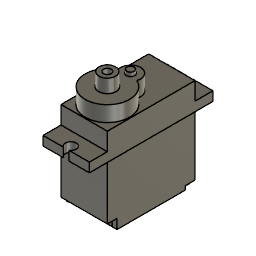
Davinki Assembly (Autodesk Fusion 360 archive; units mm, degrees)
design "Sg90Servo"
Autodesk Fusion 360 part; units mm, degrees
sketch "Sketch2" plane through (0, 0, 0) normal (0, 1, 0) x (1, 0, 0)
  line L0 (-6, -6) -> (6, -6)
  line L1 (6, -6) -> (6, 16.7)
  line L2 (6, 16.7) -> (-6, 16.7)
  line L3 (-6, 16.7) -> (-6, -6)
  line L4 (0, 0) -> (0, -6) construction
  line L5 (6, -6) -> (6, -10.65)
  line L6 (6, -10.65) -> (-6, -10.65)
  line L7 (-6, -10.65) -> (-6, -6)
  line L8 (6, 16.7) -> (6, 21.35)
  line L9 (6, 21.35) -> (-6, 21.35)
  line L10 (-6, 21.35) -> (-6, 16.7)
  line L11 (0, -10.65) -> (0, -9.45) construction
  line L12 (0, 21.35) -> (0, 20.15) construction
  circle A0 centre (0, 20.15) radius 1.4
  circle A1 centre (0, -9.45) radius 1.4
  dimension "d1" = 12
  dimension "d2" = 22.7
  dimension "d4" = 6
  dimension "d11" = 2.8
  dimension "d12" = 1.2
  dimension "d13" = 32
  constraint horizontal L0
  constraint vertical L1
  constraint horizontal L2
  constraint vertical L3
  constraint coincident L4.start origin
  constraint midpoint L0 L4.end
  constraint perpendicular L0 L4
  constraint vertical L7
  constraint horizontal L6
  constraint vertical L5
  constraint vertical L8
  constraint vertical L10
  constraint horizontal L9
  constraint equal L7 L10
  constraint midpoint L6 L11.start
  constraint perpendicular L6 L11
  constraint perpendicular L9 L12
  constraint coincident L12.end A0.centre
  constraint coincident L11.end A1.centre
  constraint equal L11 L12
  constraint equal A0 A1
  constraint midpoint L9 L12.start
  measures "d1" distance of L0.start L0.end
  measures "d2" distance of L0.start L2.end
  measures "d4" distance of L4.start L4.end
  measures "d11" diameter of A0
  measures "d12" distance of L12.start L12.end
  measures "d13" distance of L6 L9
extrude "Extrude1" add sketch "Sketch2" against normal blind 7 contours L0 L1 L2 L3 makes body 1
extrude "Extrude2" add sketch "Sketch2" along normal blind 2.4 from surface at -7 contours L0 L5 L6 L7 A1 | L2 L8 L9 L10 A0 bodies 1
extrude "Extrude3" add sketch "Sketch2" against normal blind 16.3 from surface at -7 separate body contours L0 L1 L2 L3 makes body 2
sketch "Sketch4" plane through (0, -23.3, 0) normal (0, -1, 0) x (1, 0, 0)
  line L0 (6, 6) -> (-6, 6)
  line L1 (-6, 6) -> (-6, -16.7)
  line L2 (-6, -16.7) -> (6, -16.7)
  line L3 (6, -16.7) -> (6, 6)
  circle A0 centre (4.75, -15.45) radius 1.25
  line L4 (4.75, -14.2) -> (6, -14.2)
  line L5 (3.5, -15.45) -> (3.5, -16.7)
  line L6 (-1.75, 6) -> (1.75, 6)
  line L7 (1.75, 6) -> (1.75, 4.5)
  line L8 (1.75, 4.5) -> (-1.75, 4.5)
  line L9 (-1.75, 4.5) -> (-1.75, 6)
  point P0 (0, 6)
  dimension "d20" = 2.5
  dimension "d31" = 1.5
  dimension "d32" = 3.5
  constraint tangent L3 A0
  constraint tangent L2 A0
  constraint coincident A0 L4.start
  constraint coincident L3 L4.end
  constraint tangent A0 L4
  constraint coincident A0 L5.start
  constraint coincident L2 L5.end
  constraint tangent A0 L5
  constraint perpendicular L2 L5
  constraint horizontal L4
  constraint horizontal L6
  constraint vertical L7
  constraint horizontal L8
  constraint vertical L9
  constraint midpoint L6 P0
  constraint midpoint L0 P0
  measures "d20" diameter of A0
  measures "d31" distance of L6.end L7.end
  measures "d32" distance of L7.end L8.end
ref_plane "WorkPlane1" through (0, -13.9, -5.35) normal (0, 0, 1) x (-1, 0, 0)
extrude "Extrude4" cut sketch "Sketch4" against normal blind 1 contours L3 A0 L4 | A0 | L2 L3 A0 | L2 A0 L5 bodies 2
mirror "Mirror1" about plane through (0, 0, 0) normal (1, 0, 0) of "Extrude4"
mirror "Mirror2" about plane through (0, -13.9, -5.35) normal (0, 0, 1) of "Extrude4", "Mirror1"
extrude "Extrude5" cut 2 faces at (4.75, -22.3, 4.75) (-4.75, -22.3, 4.75) along direction (0, 1, 0) blind 1.5 on bodies 2 bodies 2
chamfer "Chamfer1" distance 2.5 angle 45 1 edges at (0, -23.3, 6) tangent chain off on bodies 2
extrude "Extrude6" cut sketch "Sketch4" against normal blind 2.5 contours L0 L6 L7 L8 L9 bodies 2
sketch "Sketch3" plane through (0, 0, 0) normal (0, 1, 0) x (1, 0, 0)
  circle A0 centre (0, 0) radius 2.25
  circle A1 centre (0, 0) radius 5.75
  circle A2 centre (0, 6) radius 2.6
  line L0 (0, 6) -> (0, 0) construction
  line L1 (2.6, 6) -> (2.6, 5.1286)
  line L2 (-2.6, 6) -> (-2.6, 5.1286)
  circle A3 centre (0, 6) radius 1.1
  dimension "d5" = 4.5
  dimension "d6" = 11.5
  dimension "d7" = 5.2
  dimension "d8" = 6
  dimension "d60" = 2.2
  constraint coincident A0.centre A1.centre
  constraint coincident A2.centre L0.start
  constraint vertical L0
  constraint coincident A2 L1.start
  constraint coincident A1 L1.end
  constraint tangent A2 L1
  constraint coincident A2 L2.start
  constraint coincident A1 L2.end
  constraint tangent A2 L2
  constraint parallel L0 L2
  constraint vertical L1
  constraint concentric A2 A3
  measures "d5" diameter of A0
  measures "d6" diameter of A1
  measures "d7" diameter of A2
  measures "d8" distance of A2.centre A0.centre
  measures "d60" diameter of A3
extrude "Extrude7" add sketch "Sketch3" along normal blind 4 contours A1 A2 | A1 A2 A3 | A1 A2 A3 | A1 A3 | A1 A3 bodies 1
extrude "Extrude10" add sketch "Sketch3" along normal blind 0.9 draft -10 from surface at 4 contours A1 A3 | A1 A3 bodies 1
extrude "Extrude1'" add 1 faces at (1.1556, 0, 0.7479) along direction (0, 1, 0) blind 4 separate body on bodies 1 makes body 3 in component "Component"
extrude "Extrude2'" add 1 faces at (1.1556, 4, 0.7479) along direction (0, 1, 0) blind 3.4 draft -2 on bodies 3 bodies 3 in component "Component"
sketch "Sketch1" plane through (0, 7.4, 0) normal (0, 1, 0) x (-1, 0, 0) in component "Component"
  circle A0 centre (0, 0) radius 2.1313
  circle A1 centre (0, 0) radius 1
  dimension "d41" = 2
  constraint coincident A0.centre A1.centre
  measures "d41" diameter of A1
extrude "Extrude3'" cut sketch "Sketch1" against normal blind 3 contours A1 bodies 3 in component "Component"
sketch "Sketch5" plane through (0, -22.3, 0) normal (0, -1, 0) x (1, 0, 0)
  arc A0 (4.75, -14.2) -> (3.5, -15.45) centre (4.75, -15.45) ccw
  line L0 (3.5, -15.45) -> (3.5, -16.7)
  line L1 (3.5, -16.7) -> (6, -16.7)
  line L2 (6, -16.7) -> (6, -14.2)
  line L3 (6, -14.2) -> (4.75, -14.2)
  circle A1 centre (4.75, -15.45) radius 1
  dimension "d44" = 2
  constraint concentric A0 A1
  measures "d44" diameter of A1
extrude "Extrude8" add sketch "Sketch5" along normal blind 0.7 separate body contours A1 makes body 4
sketch "Sketch6" plane through (0, -23, 0) normal (0, -1, 0) x (1, 0, 0)
  circle A0 centre (4.75, -15.45) radius 1
  line L0 (4.5, -16.25) -> (5, -16.25)
  line L1 (5, -16.25) -> (5, -14.65)
  line L2 (5, -14.65) -> (4.5, -14.65)
  line L3 (4.5, -14.65) -> (4.5, -16.25)
  line L4 (4.5, -16.25) -> (5, -14.65) construction
  line L5 (5, -16.25) -> (4.5, -14.65) construction
  line L6 (3.95, -15.2) -> (5.55, -15.2)
  line L7 (5.55, -15.2) -> (5.55, -15.7)
  line L8 (5.55, -15.7) -> (3.95, -15.7)
  line L9 (3.95, -15.7) -> (3.95, -15.2)
  line L10 (3.95, -15.2) -> (5.55, -15.7) construction
  line L11 (5.55, -15.2) -> (3.95, -15.7) construction
  point P0 (4.75, -15.45)
  point P1 (4.75, -15.45)
  dimension "d47" = 0.5
  dimension "d48" = 1.6
  constraint horizontal L0
  constraint perpendicular L0 L1
  constraint parallel L0 L2
  constraint parallel L1 L3
  constraint coincident L4 P1
  constraint coincident L5 P1
  constraint coincident P0 A0.centre
  constraint horizontal L6
  constraint perpendicular L6 L7
  constraint parallel L6 L8
  constraint parallel L7 L9
  constraint coincident L10 P1
  constraint coincident L11 P1
  constraint coincident P1 P0
  constraint equal L0 L9
  constraint equal L3 L8
  measures "d47" distance of L6.start L8.end
  measures "d48" distance of L7.end L8.end
fillet "Fillet1" radius 0.5 1 edges at (3.8177, -23, -15.8116) on bodies 4
extrude "Extrude9" cut sketch "Sketch6" against normal blind 0.4 contours L0 L1 L3 L8 | L3 L6 L8 L9 | L1 L3 L6 L8 | L1 L6 L7 L8 | L1 L2 L3 L6 bodies 4
copy_body "CopyPasteBodies1" bodies 4 makes body 5
move_body "Move1" bodies 5 to x (1, 0, 0) y (0, 1, 0) z (0, 0, 1) at (-9.5501, 1.5, 20.1891)
sketch "Sketch7" plane through (0, -20.8, 0) normal (0, -1, 0) x (1, 0, 0)
  line L0 (-1.75, 4.5) -> (1.75, 4.5)
  line L1 (1.75, 4.5) -> (1.75, 6)
  line L2 (1.75, 6) -> (-1.75, 6)
  line L3 (-1.75, 6) -> (-1.75, 4.5)
  line L4 (0, 6) -> (0, 4.5) construction
  circle A0 centre (0, 5.25) radius 0.55
  dimension "d53" = 1.1
  constraint midpoint L2 L4.start
  constraint midpoint L0 L4.end
  constraint midpoint L4 A0.centre
  measures "d53" diameter of A0
ref_plane "WorkPlane2" through (0, -40, 0) normal (0, 1, 0) x (0, 0, 1)
sketch "Sketch8" plane through (0, -40, 0) normal (0, 1, 0) x (1, 0, 0)
  line L0 (-3.9, -4) -> (3.9, -4)
  line L1 (3.9, -4) -> (3.9, -6.8)
  line L2 (3.9, -6.8) -> (-3.9, -6.8)
  line L3 (-3.9, -6.8) -> (-3.9, -4)
  line L4 (-3.75, -4) -> (3.75, -4)
  line L5 (3.75, -4) -> (3.75, -6.5)
  line L6 (3.75, -6.5) -> (-3.75, -6.5)
  line L7 (-3.75, -6.5) -> (-3.75, -4)
  line L8 (0, -4) -> (0, -6.5) construction
  point P0 (0, -4)
  point P1 (0, -5.25)
  dimension "d65" = 2.8
  dimension "d66" = 7.8
  dimension "d67" = 2.5
  dimension "d68" = 7.5
  constraint horizontal L0
  constraint vertical L1
  constraint horizontal L2
  constraint vertical L3
  constraint horizontal L4
  constraint vertical L5
  constraint horizontal L6
  constraint vertical L7
  constraint midpoint L4 P0
  constraint midpoint L0 P0
  constraint coincident P0 L8.start
  constraint midpoint L6 L8.end
  constraint midpoint P1 L8
  measures "d65" distance of L0.end L1.end
  measures "d66" distance of L1.end L2.end
  measures "d67" distance of L4.end L5.end
  measures "d68" distance of L5.end L6.end
sketch "Sketch9" plane through (0, -49, 0) normal (0, -1, 0) x (1, 0, 0)
  line L0 (3.75, 6.5) -> (-3.75, 6.5)
  line L1 (-3.75, 6.5) -> (-3.75, 4)
  line L2 (-3.75, 4) -> (3.75, 4)
  line L3 (3.75, 4) -> (3.75, 6.5)
  line L4 (-0.5, 5.75) -> (0.5, 5.75)
  line L5 (0.5, 5.75) -> (0.5, 4.75)
  line L6 (0.5, 4.75) -> (-0.5, 4.75)
  line L7 (-0.5, 4.75) -> (-0.5, 5.75)
  line L8 (0, 4) -> (0, 6.5) construction
  line L9 (-0.5, 5.25) -> (0.5, 5.25) construction
  point P0 (0, 5.25)
  dimension "d74" = 1
  constraint horizontal L4
  constraint vertical L5
  constraint horizontal L6
  constraint vertical L7
  constraint midpoint L2 L8.start
  constraint midpoint L0 L8.end
  constraint midpoint L7 L9.start
  constraint midpoint L5 L9.end
  constraint midpoint L8 P0
  constraint midpoint L9 P0
  constraint equal L5 L6
  measures "d74" distance of L5.end L6.end
move_body "Move2" bodies 2 5 4 1 to x (1, 0, 0) y (0, 0, 1) z (0, -1, 0) at (0, -37.725, 7.875)
move_body "Move1'" bodies 3 to x (1, 0, 0) y (0, 0, 1) z (0, -1, 0) at (0, -37.725, 7.875) in component "Component"
move_body "Move3" bodies 5 2 4 1 to x (1, 0, 0) y (0, 1, 0) z (0, 0, 1) at (0, 40, 16)
move_body "Move2'" bodies 3 to x (1, 0, 0) y (0, 1, 0) z (0, 0, 1) at (0, 40, 16) in component "Component"
component "Component" placed x (1, 0, 0) y (0, 1, 0) z (0, 0, 1) at (0, 0, 0)
equation "d18 = 7 mm - 23.3 mm"

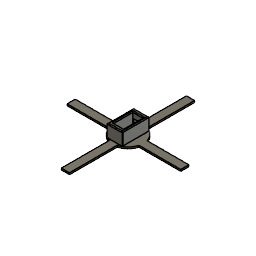
design "Davinki Base"
part number: 2026-08-29-10-07-06-773
Autodesk Fusion 360 part; units mm, degrees
sketch "Sketch1" plane through (0, 0, 0) normal (0, 1, 0) x (1, 0, 0)
  line L0 (0, 0) -> (12.25, 0)
  line L1 (12.25, 0) -> (12.25, 23.5)
  line L2 (0, 0) -> (0, 23.5)
  line L3 (0, 23.5) -> (12.25, 23.5)
  line L4 (-3.4056, 0) -> (-3.4056, 27)
  line L5 (-3.4056, 27) -> (15.0988, 27)
  line L6 (15.0988, 27) -> (15.0988, -3.5)
  line L7 (15.0988, -3.5) -> (-3.4056, -3.5)
  line L8 (-3.4056, -3.5) -> (-3.4056, 27)
  line L9 (-3.4056, 27) -> (-3.4056, 28)
  line L10 (-3.4056, 28) -> (15.0988, 28)
  line L11 (15.0988, 28) -> (15.0988, 27)
  line L12 (-3.4056, -3.5) -> (-3.4056, -4.5)
  line L13 (-3.4056, -4.5) -> (15.1, -4.5)
  line L14 (15.1, -4.5) -> (15.0988, -3.5)
  line L15 (0, 23.5) -> (0, 0.25)
  line L16 (5.8472, -4.5) -> (5.8472, -29.5)
  line L17 (5.8472, -29.5) -> (10.8472, -29.5)
  line L18 (10.8472, -29.5) -> (0.8472, -29.5)
  line L19 (0.8472, -29.5) -> (0.8472, -4.5)
  line L20 (10.8472, -29.5) -> (10.8472, -4.5)
  line L21 (5.8466, 28) -> (5.8466, 53)
  line L22 (5.8466, 53) -> (10.8466, 53)
  line L23 (10.8466, 53) -> (0.8466, 53)
  line L24 (0.8466, 53) -> (0.8466, 28)
  line L25 (10.8466, 53) -> (10.8466, 28)
  line L26 (12.25, 11.75) -> (-3.4056, 11.75)
  line L27 (-3.4056, 11.75) -> (-28.4056, 11.75)
  line L28 (-28.4056, 11.75) -> (-28.4056, 6.75)
  line L29 (-28.4056, 6.75) -> (-28.4056, 16.75)
  line L30 (-28.4056, 16.75) -> (-3.4056, 16.7633)
  line L31 (-28.4056, 6.75) -> (-3.4056, 6.75)
  line L32 (15.0988, 11.75) -> (40.0988, 11.75)
  line L33 (40.0988, 11.75) -> (40.0988, 6.75)
  line L34 (40.0988, 6.75) -> (40.0988, 16.75)
  line L35 (40.0988, 16.75) -> (15.0988, 16.75)
  line L36 (40.0988, 6.75) -> (15.0988, 6.75)
  line L37 (-28.4056, 16.75) -> (-63.4056, 16.75)
  line L38 (-28.4056, 6.75) -> (-63.4056, 6.75)
  line L39 (-63.4056, 6.75) -> (-63.4056, 16.75)
  line L40 (40.0988, 16.75) -> (75.0988, 16.75)
  line L41 (75.0988, 16.75) -> (75.0988, 6.75)
  line L42 (75.0988, 6.75) -> (40.0988, 6.75)
  line L43 (10.8466, 53) -> (10.8466, 88)
  line L44 (0.8466, 53) -> (0.8466, 88)
  line L45 (0.8466, 88) -> (10.8466, 88)
  line L46 (10.8472, -29.5) -> (10.8472, -64.5)
  line L47 (10.8472, -64.5) -> (0.8466, -64.5)
  line L48 (0.8466, -64.5) -> (0.8472, -29.5)
  circle A0 centre (5.9954, 11.75) radius 18.8312
  dimension "d1" = 12.25
  dimension "d2" = 23.5
  dimension "d3" = 23.5
  dimension "d6" = 30.5
  dimension "d7" = 1
  dimension "d8" = 1
  dimension "d16" = 23.25
  dimension "d17" = 25
  dimension "d18" = 5
  dimension "d19" = 10
  dimension "d20" = 25
  dimension "d21" = 5
  dimension "d22" = 10
  dimension "d23" = 25
  dimension "d24" = 5
  dimension "d25" = 10
  dimension "d26" = 25
  dimension "d30" = 25
  dimension "d31" = 5
  dimension "d32" = 10
  dimension "d35" = 35
  dimension "d36" = 35
  dimension "d37" = 35
  dimension "d38" = 35
  dimension "d39" = 35
  dimension "d40" = 35
  constraint coincident L0.start L2.start
  constraint horizontal L0
  constraint perpendicular L0 L1
  constraint perpendicular L0 L2
  constraint horizontal L5
  constraint vertical L6
  constraint horizontal L7
  constraint vertical L8
  constraint perpendicular L5 L9
  constraint perpendicular L6 L10
  constraint perpendicular L5 L11
  constraint perpendicular L7 L12
  constraint perpendicular L8 L13
  constraint perpendicular L0 L15
  constraint midpoint L13 L16.start
  constraint perpendicular L13 L16
  constraint perpendicular L16 L17
  constraint perpendicular L16 L18
  constraint coincident L13 L19.end
  constraint perpendicular L13 L19
  constraint perpendicular L17 L20
  constraint midpoint L10 L21.start
  constraint perpendicular L10 L21
  constraint perpendicular L21 L22
  constraint perpendicular L21 L23
  constraint coincident L10 L24.end
  constraint perpendicular L10 L24
  constraint coincident L10 L25.end
  constraint perpendicular L10 L25
  constraint midpoint L1 L26.start
  constraint midpoint L8 L26.end
  constraint perpendicular L4 L26
  constraint perpendicular L8 L27
  constraint perpendicular L27 L28
  constraint perpendicular L27 L29
  constraint coincident L8 L30.end
  constraint perpendicular L8 L31
  constraint midpoint L6 L32.start
  constraint perpendicular L6 L32
  constraint perpendicular L32 L33
  constraint perpendicular L32 L34
  constraint coincident L6 L35.end
  constraint perpendicular L6 L35
  constraint coincident L6 L36.end
  constraint perpendicular L6 L36
  constraint perpendicular L29 L37
  constraint perpendicular L28 L38
  constraint perpendicular L34 L40
  constraint perpendicular L35 L41
  constraint perpendicular L34 L42
  constraint perpendicular L42 L43
  constraint perpendicular L23 L44
  constraint perpendicular L43 L45
  constraint perpendicular L18 L46
  constraint perpendicular L20 L47
  constraint coincident L26 A0.centre
  measures "d1" distance of L0.start L0.end
  measures "d2" distance of L0.end L1.end
  measures "d3" distance of L0.start L2.end
  measures "d6" distance of L4.end L7.end
  measures "d7" distance of L4.end L9.end
  measures "d8" distance of L7.end L12.end
  measures "d16" distance of L2.end L15.end
  measures "d17" distance of L16.start L16.end
  measures "d18" distance of L16.end L17.end
  measures "d19" distance of L17.end L18.end
  measures "d20" distance of L21.start L21.end
  measures "d21" distance of L21.end L22.end
  measures "d22" distance of L22.end L23.end
  measures "d23" distance of L26.end L27.end
  measures "d24" distance of L27.end L28.end
  measures "d25" distance of L28.end L29.end
  measures "d26" distance of L28.end L31.end
  measures "d30" distance of L32.start L32.end
  measures "d31" distance of L32.end L33.end
  measures "d32" distance of L33.end L34.end
  measures "d35" distance of L29.end L37.end
  measures "d36" distance of L28.end L38.end
  measures "d37" distance of L34.end L40.end
  measures "d38" distance of L22.end L43.end
  measures "d39" distance of L23.end L44.end
  measures "d40" distance of L17.end L46.end
extrude "Extrude1" add sketch "Sketch1" along normal blind 17.3 contours L4 L5 L6 L7 L8 | L7 L12 L13 L14 | L5 L9 L10 L11
sketch "Sketch2" plane through (0, 0, -28) normal (0, 0, -1) x (-1, 0, 0)
  line L0 (-15.0988, 0) -> (3.4056, 0)
  line L1 (3.4056, 0) -> (3.4056, 17.3)
  line L2 (3.4056, 17.3) -> (-15.0988, 17.3)
  line L3 (-15.0988, 17.3) -> (-15.0988, 0)
  line L4 (-11.5, 2) -> (-1.0253, 2)
  line L5 (-1.0253, 2) -> (-1.0253, 5)
  line L6 (-11.5, 5) -> (-11.5, 2)
  line L7 (-11.5, 5) -> (-11.5, 10)
  line L8 (-11.5, 10) -> (-1, 10)
  line L9 (-1, 10) -> (-1.0253, 5)
  dimension "d11" = 3
  constraint horizontal L4
  constraint vertical L5
  constraint vertical L6
  constraint perpendicular L7 L8
  measures "d11" distance of L4.start L6.start
extrude "Extrude2" cut sketch "Sketch2" against normal blind 16 contours L4 L5 L6 L7 L8 L9
fillet "Fillet1" radius 1 1 faces at (3.8981, 17.3, 3)
extrude "Extrude3" add sketch "Sketch1" along normal blind 2 contours L4 L8 L27 L31 A0 | L4 L8 L27 L30 A0 | L27 L28 L29 L31 A0 | L27 L29 L30 A0 | L16 L18 L19 A0 | L13 L16 L19 A0 | L6 L32 L36 A0 | L16 L17 L18 L20 A0 | L13 L16 L20 A0 | L6 L32 L35 A0 | L32 L33 L34 L36 A0 | L10 L21 L24 A0 | L21 L23 L24 A0 | L32 L34 L35 A0 | L10 L21 L25 A0 | L21 L22 L23 L25 A0
extrude "Extrude4" add sketch "Sketch1" along normal blind 2 contours L28 L29 L37 L38 L39 | L17 L18 L46 L47 L48 | L33 L34 L40 L41 L42 | L22 L23 L43 L44 L45
extrude "Extrude5" add sketch "Sketch1" along normal blind 2 contours L4 L8 L12 L13 L19 L31 A0 | L6 L13 L14 L20 L36 A0 | L4 L8 L9 L10 L24 L30 A0 | L6 L10 L11 L25 L35 A0
